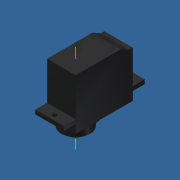
# Autodesk Inventor part: Servo G12DM
Saved by Autodesk Inventor 2016 (Build 200138000, 138)
## iProperties
Created: 2013-10-15
Part Number: Servo G12DM
Material: ABS-Kunststoff - Schwarz
Document SubType Name: Modeling
Designer: 4ndreas
Density: 1.06 g/cm^3
Appearance: Glatt - weiß(2)
Mass: 7.06899 g
Surface Area: 25.6588 cm^2
Volume: 6.66886 cm^3
Author: 4ndreas
Autodesk Inventor part; units mm, degrees
ref_plane "YZ Plane" through (0, 0, 0) normal (1, 0, 0) x (0, 1, 0)
ref_plane "XZ Plane" through (0, 0, 0) normal (0, 1, 0) x (-1, 0, 0)
ref_plane "XY Plane" through (0, 0, 0) normal (0, 0, 1) x (1, 0, 0)
sketch "Skizze1" plane through (0, 0, 0) normal (0, 0, 1) x (1, 0, 0)
  line L0 (0.0823, -4.147) -> (0.0823, -9.8981)
  line L1 (0.0823, -9.8981) -> (-11.9177, -9.8981)
  line L2 (-11.9177, -9.8981) -> (-11.9177, 14.1019)
  line L3 (-11.9177, 14.1019) -> (0.0823, 14.1019)
  line L4 (0.0823, 14.1019) -> (0.0823, -4.147)
  point P0 (0, 0)
  dimension "d34" = 12
  dimension "d35" = 24
  constraints: 10 end point, 2 perpendicular, 1 collinear
  measures "d34" distance between parallel lines of L0 L2
  measures "d35" distance between parallel lines of L1 L3
extrude "Extrusion1" add sketch "Skizze1" against normal blind 3.6
sketch "Skizze2" plane through (0, 0, 0) normal (0, 0, 1) x (1, 0, 0)
  line L0 (0.0823, -9.8981) -> (0.0823, 14.1019) projected
  line L1 (0.0823, 14.1019) -> (-11.9177, 14.1019) projected
  line L2 (-11.9177, 14.1019) -> (-11.9177, -9.8981) projected
  line L3 (-11.9177, -9.8981) -> (0.0823, -9.8981) projected
  line L4 (-11.9177, 19.1019) -> (0.0823, 19.1019)
  line L5 (0.0823, 19.1019) -> (0.0823, -14.8981)
  line L6 (0.0823, -14.8981) -> (-11.9177, -14.8981)
  line L7 (-11.9177, -14.8981) -> (-11.9177, 19.1019)
  point P0 (0, 0)
  dimension "d2" = 5
  dimension "d3" = 5
  constraints: 8 end point, 2 collinear, 2 parallel, 1 horizontal, 1 perpendicular
  measures "d2" distance between parallel lines of L1 L4
  measures "d3" distance between parallel lines of L6 L3
extrude "Extrusion2" add sketch "Skizze2" along normal blind 1.7
sketch "Skizze3" plane through (0, 0, 1.7) normal (0, 0, 1) x (1, 0, 0)
  line L0 (0.0823, 14.1019) -> (0.0823, -9.8981) projected
  line L1 (0.0823, -9.8981) -> (-11.9177, -9.8981) projected
  line L2 (-11.9177, -9.8981) -> (-11.9177, 14.1019) projected
  line L3 (-11.9177, 14.1019) -> (0.0823, 14.1019) projected
  point P0 (0, 0)
extrude "Extrusion3" add sketch "Skizze3" along normal blind 16
sketch "Skizze4" plane through (0, 0, -3.6) normal (0, 0, -1) x (-1, 0, 0)
  line L0 (-0.0823, -9.8981) -> (11.9177, -9.8981) projected
  line L1 (11.9177, 14.1019) -> (-0.0823, 14.1019) projected
  circle A0 centre (5.9177, -3.8981) radius 6
  line L2 (5.9177, 14.1019) -> (5.9177, -9.8981) construction
  line L3 (5.9177, -3.8981) -> (5.9177, 1.8519) construction
  line L4 (9.1677, -3.8981) -> (9.1677, 1.8519)
  line L5 (2.6677, 1.8519) -> (2.6677, -3.8981)
  arc A1 (2.6677, -3.8981) -> (9.1677, -3.8981) centre (5.9177, -3.8981) ccw
  arc A2 (9.1677, 1.8519) -> (2.6677, 1.8519) centre (5.9177, 1.8519) ccw
  line L6 (-0.0823, 14.1019) -> (-0.0823, -9.8981) projected
  point P0 (0, 0)
  point P1 (5.9177, -1.0231)
  dimension "d32" = 6.5
  dimension "d33" = 15
  constraints: 10 end point, 6 tangent, 4 point on circle, 3 centre point, 3 midpoint, 2 point on line, 1 parallel
  measures "d32" distance between parallel lines of L4 L5
extrude "Extrusion4" add sketch "Skizze4" along normal blind 3 contours A0 L5 A1 L4 | L5 A2 L4 A0 | A0 L4 A1 L5
sketch "Skizze5" plane through (0, 0, -3.6) normal (0, 0, -1) x (-1, 0, 0)
  circle A0 centre (5.9177, -3.8981) radius 6 projected
  line L0 (-0.0823, 14.1019) -> (-0.0823, -9.8981) projected
  line L1 (-0.0823, -9.8981) -> (11.9177, -9.8981) projected
  line L2 (11.9177, -9.8981) -> (11.9177, 14.1019) projected
  line L3 (11.9177, 14.1019) -> (-0.0823, 14.1019) projected
  point P0 (0, 0)
sketch "Skizze7" plane through (0, 0, 0) normal (0, 0, -1) x (-1, 0, 0)
  line L0 (-0.0823, -9.8981) -> (-0.0823, -14.8981) projected
  line L1 (-0.0823, -14.8981) -> (11.9177, -14.8981) projected
  line L2 (-0.0823, 14.1019) -> (11.9177, 14.1019) projected
  line L3 (11.9177, 14.1019) -> (11.9177, 19.1019) projected
  line L4 (11.9177, 19.1019) -> (-0.0823, 19.1019) projected
  line L5 (-0.0823, 19.1019) -> (-0.0823, 14.1019) projected
  point P0 (0, 0)
  point P1 (5.9177, 17.1019)
  point P2 (5.9177, -12.8981)
  dimension "d12" = 2
  dimension "d13" = 2
  dimension "d14" = 12
  dimension "d15" = 6
  dimension "d16" = 6
  measures "d12" distance from line of L4 point (5.918, 17.102)
  measures "d13" distance from line of point (5.918, -12.898) L1
  measures "d14" distance between parallel lines of L3 L5
  measures "d15" distance from line of L5 point (5.918, 17.102)
  measures "d16" distance from line of L0 point (5.918, -12.898)
hole "Bohrung1" at (-5.9177, -12.8981, 0) at (-5.9177, 17.1019, 0) direction (0, 0, 1) diameter 1.7 end through all
sketch "Skizze9" plane through (0, 0, -6.6) normal (0, 0, -1) x (-1, 0, 0)
  arc A0 (2.6677, 1.1454) -> (9.1677, 1.1454) centre (5.9177, -3.8981) ccw projected
  circle A1 centre (5.9177, -3.8981) radius 1.85
  point P0 (0, 0)
  dimension "d36" = 3.7
  constraints: 1 centre point, 1 coincident
  measures "d36" diameter of A1
extrude "Extrusion6" add sketch "Skizze9" along normal blind 3.5 separate body
chamfer "Fase1" distance 0.2 angle 45 1 edges at (-4.0677, -3.8981, -10.1)
sketch "Skizze10" plane through (0.0823, 14.1019, 0) normal (1, 0, 0) x (0, 0, -1)
  line L0 (-1.7, 0) -> (-17.7, 0) projected
  line L1 (-17.7, -24) -> (-17.7, 0) projected
  line L2 (0, -24) -> (0, -29) projected
  line L3 (-15.7, 0) -> (-15.7, -1.5359)
  line L4 (-15.7, -1.5359) -> (-17.7, -5)
  point P0 (0, -14.1019)
  dimension "d42" = 30
  dimension "d43" = 2
  dimension "d44" = 5
  constraints: 4 end point, 2 point on line, 1 parallel
  measures "d42" angle of L1 L4
  measures "d43" distance between parallel lines of L1 L3
  measures "d44" distance from line of L4.end L0
extrude "Extrusion7" cut sketch "Skizze10" against normal through all bodies 1
hole "Bohrung2" at (-5.9177, -3.8981, -10.1) direction (0, 0, 1) diameter 2 depth 5 tip angle 118 bodies 2
equation "\"d15\" = 0.5 * d14"
equation "\"d16\" = d15"
